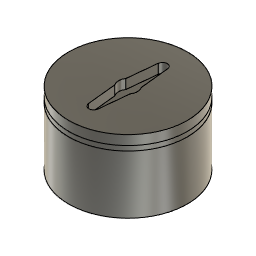
servo_double v2 (Autodesk Fusion 360 archive; units mm, degrees)
design "servo"
Autodesk Fusion 360 part; units mm, degrees
sketch "スケッチ1" plane through (0, 0, 0) normal (0, 0, 1) x (1, 0, 0)
  circle A0 centre (0, 0) radius 25
  line L0 (3.2646, -2.3114) -> (1.9895, -14.7047)
  line L1 (-3.2646, -2.3114) -> (-1.9895, -14.7047)
  line L2 (-3.2597, 2.3182) -> (-1.9896, 14.704)
  arc A1 (1.9896, 14.704) -> (-1.9896, 14.704) centre (0, 14.5) ccw
  arc A2 (-1.9895, -14.7047) -> (1.9895, -14.7047) centre (0, -14.5) ccw
  line L3 (3.2597, 2.3182) -> (1.9896, 14.704)
  arc A3 (3.2646, -2.3114) -> (3.2597, 2.3182) centre (0, 0) ccw
  arc A4 (-3.2597, 2.3182) -> (-3.2646, -2.3114) centre (0, 0) ccw
  dimension "d1" = 50
  dimension "d3" = 4
  dimension "d5" = 4
  dimension "d7" = 8
  constraint coincident A0.centre A3.centre
  constraint tangent L0 A2
  constraint tangent L1 A2
  constraint tangent L2 A1
  constraint coincident L2.start A3
  constraint concentric A3 A4
  measures "d1" diameter of A0
  measures "d3" diameter of A1
  measures "d5" diameter of A2
  measures "d7" diameter of A3
extrude "押し出し1" add sketch "スケッチ1" along normal blind 4 makes body 1
sketch "スケッチ2" plane through (0, 0, 4) normal (0, 0, 1) x (-1, 0, 0)
  arc A0 (-3.2646, 2.3114) -> (-3.2597, -2.3182) centre (0, 0) ccw
  line L0 (-3.2646, 2.3114) -> (-1.9895, 14.7047)
  arc A1 (1.9895, 14.7047) -> (-1.9895, 14.7047) centre (0, 14.5) ccw
  line L1 (1.9895, 14.7047) -> (3.2646, 2.3114)
  arc A2 (3.2597, -2.3182) -> (3.2646, 2.3114) centre (0, 0) ccw
  line L2 (3.2597, -2.3182) -> (1.9896, -14.704)
  arc A3 (-1.9896, -14.704) -> (1.9896, -14.704) centre (0, -14.5) ccw
  line L3 (-1.9896, -14.704) -> (-3.2597, -2.3182)
  circle A4 centre (0, 0) radius 25
  circle A5 centre (55, 0) radius 25
  dimension "d10" = 50
  measures "d10" diameter of A5
extrude "押し出し2" add sketch "スケッチ2" along normal blind 2 separate body contours A5 makes body 2
move_body "移動1" bodies 2 to x (1, 0, 0) y (0, 1, 0) z (0, 0, 1) at (55, 0, -6)
extrude "押し出し3" cut 1 faces at (-7.8601, -11.3401, 4) along direction (0, 0, -1) blind 1 on bodies 1 bodies 1
sketch "スケッチ3" plane through (0, 0, 3) normal (0, 0, 1) x (-1, 0, 0)
  arc A0 (-3.2646, 2.3114) -> (-3.2597, -2.3182) centre (0, 0) ccw
  line L0 (-3.2646, 2.3114) -> (-1.9895, 14.7047)
  arc A1 (1.9895, 14.7047) -> (-1.9895, 14.7047) centre (0, 14.5) ccw
  line L1 (1.9895, 14.7047) -> (3.2646, 2.3114)
  arc A2 (3.2597, -2.3182) -> (3.2646, 2.3114) centre (0, 0) ccw
  line L2 (3.2597, -2.3182) -> (1.9896, -14.704)
  arc A3 (-1.9896, -14.704) -> (1.9896, -14.704) centre (0, -14.5) ccw
  line L3 (-1.9896, -14.704) -> (-3.2597, -2.3182)
  circle A4 centre (0, 0) radius 25
  circle A5 centre (-74.9851, 0.0123) radius 25
  line L4 (-97.2842, -2.9877) -> (-80.9851, -2.9877)
  line L5 (-77.9851, -5.9877) -> (-77.9851, -22.2869)
  line L6 (-52.686, 3.0123) -> (-68.9851, 3.0123)
  line L7 (-71.9851, 6.0123) -> (-71.9851, 22.3114)
  arc A6 (-77.9851, -5.9877) -> (-80.9851, -2.9877) centre (-80.9851, -5.9877) ccw
  arc A7 (-71.9851, 6.0123) -> (-68.9851, 3.0123) centre (-68.9851, 6.0123) ccw
  arc A8 (-77.9851, -22.2869) -> (-52.686, 3.0123) centre (-74.9851, 0.0123) ccw
  arc A9 (-71.9851, 22.3114) -> (-97.2842, -2.9877) centre (-74.9851, 0.0123) ccw
  dimension "d15" = 50
  dimension "d16" = 45
  dimension "d19" = 6
  dimension "d20" = 6
  dimension "d21" = 3
  dimension "d22" = 3
  dimension "d23" = 3
  dimension "d24" = 3
  constraint concentric A5 A8
  constraint horizontal L4
  constraint vertical L5
  constraint horizontal L6
  constraint vertical L7
  constraint tangent L5 A6
  constraint tangent L4 A6
  constraint tangent L6 A7
  constraint tangent L7 A7
  constraint concentric A8 A9
  measures "d15" diameter of A5
  measures "d16" diameter of A8
  measures "d19" distance of L4 L6
  measures "d20" distance of L5 L7
  measures "d21" distance of A5.centre L4
  measures "d22" distance of A5.centre L5
  measures "d23" radius of A6
  measures "d24" radius of A7
extrude "押し出し4" add sketch "スケッチ3" along normal blind 10 separate body contours A5 makes body 3
extrude "押し出し5" add 1 faces at (-7.8601, -11.3401, 3) along direction (0, 0, 1) blind 1 on bodies 1 bodies 1
move_body "移動2" bodies 1 2 to x (1, 0, 0) y (0, 1, 0) z (0, 0, 1) at (75, 0, 15)
move_body "移動3" bodies 3 1 2 to x (1, 0, 0) y (0, 1, 0) z (0, 0, 1) at (-75, 0, 0)
sketch "スケッチ4" plane through (0, 0, 3) normal (0, 0, -1) x (1, 0, 0)
  line L0 (-3.0149, 6.0123) -> (-3.0149, 22.3114)
  arc A0 (22.2842, -2.9877) -> (-3.0149, 22.3114) centre (-0.0149, 0.0123) ccw
  line L1 (22.2842, -2.9877) -> (5.9851, -2.9877)
  arc A1 (5.9851, -2.9877) -> (2.9851, -5.9877) centre (5.9851, -5.9877) ccw
  line L2 (2.9851, -5.9877) -> (2.9851, -22.2869)
  arc A2 (-22.314, 3.0123) -> (2.9851, -22.2869) centre (-0.0149, 0.0123) ccw
  line L3 (-22.314, 3.0123) -> (-6.0149, 3.0123)
  arc A3 (-6.0149, 3.0123) -> (-3.0149, 6.0123) centre (-6.0149, 6.0123) ccw
  circle A4 centre (-0.0149, 0.0123) radius 25
  circle A5 centre (-0.0149, 0.0123) radius 25
  circle A6 centre (-0.0149, 0.0123) radius 22.5
  dimension "d29" = 50
  dimension "d30" = 45
  constraint concentric A0 A5
  constraint concentric A5 A6
  measures "d29" diameter of A5
  measures "d30" diameter of A6
extrude "押し出し6" add sketch "スケッチ4" along normal blind 15 bodies 3
move_body "移動4" bodies 1 2 3 to x (1, 0, 0) y (0, 1, 0) z (0, 0, 1) at (0, 0, 12)
sketch "スケッチ5" plane through (0, 0, 0) normal (0, 1, 0) x (1, 0, 0)
extrude "押し出し7" cut 1 faces at (-3.606, 23.839, 0) along direction (0, 0, 1) blind 0.5 on bodies 3 bodies 3

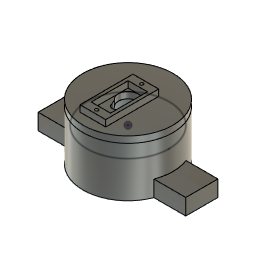
design "servo_up"
Autodesk Fusion 360 part; units mm, degrees
sketch "スケッチ1" plane through (0, 0, 0) normal (0, 0, 1) x (1, 0, 0)
  circle A0 centre (0, 0) radius 25.5
  circle A1 centre (0, 0) radius 22.5
  circle A2 centre (0, 0) radius 28
  dimension "d1" = 51
  dimension "d2" = 45
  dimension "d3" = 56
  constraint coincident A0.centre A1.centre
  constraint concentric A0 A2
  measures "d1" diameter of A0
  measures "d2" diameter of A1
  measures "d3" diameter of A2
extrude "押し出し1" add sketch "スケッチ1" along normal blind 25 contours A2 makes body 1
sketch "スケッチ2" plane through (0, 0, 0) normal (0, 0, 1) x (1, 0, 0)
  circle A0 centre (0, 0) radius 22.5
  circle A1 centre (0, 0) radius 25.5
  dimension "d6" = 45
  dimension "d7" = 51
  constraint coincident A0.centre A1.centre
  measures "d6" diameter of A0
  measures "d7" diameter of A1
extrude "押し出し2" add sketch "スケッチ2" along normal blind 15 bodies 1
sketch "スケッチ3" plane through (0, 0, 0) normal (0, 0, 1) x (1, 0, 0)
  line L0 (-31.9093, 14.985) -> (-51.9093, 14.985)
  line L1 (-51.9093, 14.985) -> (-51.9093, -15.015)
  line L2 (-51.9093, -15.015) -> (-31.9093, -15.015)
  line L3 (-31.9093, -15.015) -> (-31.9093, 14.985)
  circle A0 centre (-41.9093, -0.0927) radius 7
  dimension "d10" = 20
  dimension "d11" = 30
  dimension "d12" = 14
  dimension "d13" = 10
  constraint horizontal L0
  constraint vertical L1
  constraint horizontal L2
  constraint vertical L3
  measures "d10" distance of L0.start L0.end
  measures "d11" distance of L0.end L1.end
  measures "d12" diameter of A0
  measures "d13" distance of L1 A0.centre
sketch "スケッチ4" plane through (0, 0, 0) normal (0, 0, 1) x (1, 0, 0)
sketch "スケッチ5" plane through (0, 0, 0) normal (0, 1, 0) x (1, 0, 0)
sketch "スケッチ6" plane through (0, 0, 0) normal (0, 0, 1) x (1, 0, 0)
  line L0 (-60, 20) -> (-40, 20)
  line L1 (-40, 20) -> (-40, 0)
  line L2 (-40, 0) -> (-60, 0)
  line L3 (-60, 0) -> (-60, 20)
  dimension "d16" = 20
  constraint horizontal L0
  constraint vertical L1
  constraint horizontal L2
  constraint vertical L3
  measures "d16" distance of L0.start L0.end
extrude "押し出し4" add sketch "スケッチ6" along normal blind 10 separate body makes body 2
sketch "スケッチ7" plane through (0, 0, 0) normal (0, 0, 1) x (1, 0, 0)
  circle A0 centre (-50, 10) radius 7
  dimension "d19" = 14
  measures "d19" diameter of A0
extrude "押し出し5" cut sketch "スケッチ7" along normal blind 2.5 bodies 2
copy_body "ボディのコピーと貼り付け1" bodies 2 makes body 3
sketch "スケッチ8" plane through (0, 0, 0) normal (0, 0, 1) x (1, 0, 0)
  line L0 (35, 20) -> (55, 20)
  line L1 (55, 20) -> (55, 0)
  line L2 (55, 0) -> (35, 0)
  line L3 (35, 0) -> (35, 20)
  dimension "d22" = 20
  constraint horizontal L0
  constraint vertical L1
  constraint horizontal L2
  constraint vertical L3
  measures "d22" distance of L0.start L0.end
extrude "押し出し6" add sketch "スケッチ8" along normal blind 10 separate body makes body 4
sketch "スケッチ9" plane through (0, 0, 0) normal (0, 0, 1) x (1, 0, 0)
  circle A0 centre (45, 10) radius 7
  dimension "d25" = 14
  measures "d25" diameter of A0
extrude "押し出し7" cut sketch "スケッチ9" along normal blind 2.5 bodies 4
move_body "移動1" bodies 3 2 to x (1, 0, 0) y (0, 1, 0) z (0, 0, 1) at (0, -20, 0)
move_face "面を移動1" by (0, 10, 0) 1 faces at (-53.3333, -6.6667, 10) on bodies 3
move_body "移動2" bodies 2 3 to x (1, 0, 0) y (0, 1, 0) z (0, 0, 1) at (0, 10, 0)
move_body "移動3" bodies 2 3 to x (1, 0, 0) y (0, 1, 0) z (0, 0, 1) at (14, 0, 0)
move_body "移動4" bodies 4 to x (1, 0, 0) y (0, 1, 0) z (0, 0, 1) at (-9, -10, 0)
sketch "スケッチ10" plane through (0, 0, 0) normal (0, 0, 1) x (1, 0, 0)
  line L0 (70, 15) -> (140, 15)
  line L1 (140, 15) -> (140, -23)
  line L2 (140, -23) -> (70, -23)
  line L3 (70, -23) -> (70, 15)
  line L4 (90, 0) -> (113, 0)
  line L5 (113, 0) -> (113, -12)
  line L6 (113, -12) -> (90, -12)
  line L7 (90, -12) -> (90, 0)
  dimension "d28" = 70
  dimension "d29" = 23
  dimension "d30" = 12
  dimension "d31" = 38
  constraint horizontal L0
  constraint vertical L1
  constraint horizontal L2
  constraint vertical L3
  constraint horizontal L4
  constraint vertical L5
  constraint horizontal L6
  constraint vertical L7
  measures "d28" distance of L0.start L0.end
  measures "d29" distance of L4.start L4.end
  measures "d30" distance of L4 L6
  measures "d31" distance of L0.end L1.end
sketch "スケッチ11" plane through (0, 0, 0) normal (0, 0, 1) x (1, 0, 0)
  line L0 (113, -12) -> (118, -12)
  line L1 (118, -12) -> (118, 0)
  line L2 (118, 0) -> (113, 0)
  line L3 (113, 0) -> (113, -12)
  line L4 (90, -12) -> (85, -12)
  line L5 (85, -12) -> (85, 0)
  line L6 (85, 0) -> (90, 0)
  line L7 (90, 0) -> (90, -12)
  dimension "d34" = 5
  dimension "d35" = 5
  dimension "d36" = 12
  dimension "d37" = 12
  constraint horizontal L0
  constraint vertical L1
  constraint horizontal L2
  constraint vertical L3
  constraint horizontal L4
  constraint vertical L5
  constraint horizontal L6
  constraint vertical L7
  measures "d34" distance of L0.start L0.end
  measures "d35" distance of L4.start L4.end
  measures "d36" distance of L0 L2
  measures "d37" distance of L4 L6
sketch "スケッチ12" plane through (0, 0, 0) normal (0, 0, 1) x (1, 0, 0)
  circle A0 centre (-102, 0) radius 28
  line L0 (-99.5001, -7.5215) -> (-99.4823, -5.4462)
  line L1 (-104.5, -7.5) -> (-104.5, -5.4544)
  arc A1 (-104.5, -7.5) -> (-99.5001, -7.5215) centre (-102, -7.5) ccw
  arc A2 (-99.4823, -5.4462) -> (-104.5, -5.4544) centre (-102, 0) ccw
  dimension "d40" = 56
  dimension "d41" = 12
  dimension "d42" = 5
  dimension "d43" = 7.5
  constraint concentric A0 A2
  constraint tangent L0 A1
  constraint tangent L1 A1
  constraint vertical L1
  measures "d40" diameter of A0
  measures "d41" diameter of A2
  measures "d42" diameter of A1
  measures "d43" distance of A0.centre A1.centre
extrude "押し出し10" add sketch "スケッチ12" along normal blind 5 separate body makes body 5
sketch "スケッチ13" plane through (0, 0, 15) normal (0, 0, 1) x (-1, 0, 0)
  circle A0 centre (0, 0) radius 22.5
  circle A1 centre (0, 0) radius 25.5
sketch "スケッチ14" plane through (0, 0, 15) normal (0, 0, 1) x (1, 0, 0)
  circle A0 centre (0, 0) radius 25.5
  dimension "d46" = 51
  constraint coincident A0.centre origin
  measures "d46" diameter of A0
sketch "スケッチ15" plane through (0, 0, 15) normal (0, 0, 1) x (1, 0, 0)
sketch "スケッチ16" plane through (0, 0, 15) normal (0, 0, 1) x (1, 0, 0)
  line L0 (-108, 6.0876) -> (-96, 6.0876)
  line L1 (-96, 6.0876) -> (-96, -16.9124)
  line L2 (-96, -16.9124) -> (-108, -16.9124)
  line L3 (-108, -16.9124) -> (-108, 6.0876)
  line L4 (-110, 11.0876) -> (-94, 11.0876)
  line L5 (-94, 11.0876) -> (-94, -21.9124)
  line L6 (-94, -21.9124) -> (-110, -21.9124)
  line L7 (-110, -21.9124) -> (-110, 11.0876)
  dimension "d47" = 12
  dimension "d48" = 23
  dimension "d50" = 5
  dimension "d51" = 5
  dimension "d52" = 2
  dimension "d53" = 2
  constraint horizontal L0
  constraint vertical L1
  constraint horizontal L2
  constraint vertical L3
  constraint horizontal L4
  constraint vertical L5
  constraint horizontal L6
  constraint vertical L7
  measures "d47" distance of L1 L3
  measures "d48" distance of L0 L2
  measures "d50" distance of L2 L6
  measures "d51" distance of L0 L4
  measures "d52" distance of L1 L5
  measures "d53" distance of L3 L7
extrude "押し出し11" add sketch "スケッチ16" along normal blind 7 separate body makes body 6
move_body "移動5" bodies 6 to x (1, 0, 0) y (0, 1, 0) z (0, 0, 1) at (0, 0, -10)
extrude "押し出し12" cut 1 faces at (-92.8319, -10.3859, 0) along direction (0, 0, 1) blind 1 on bodies 5 bodies 5
extrude "押し出し13" cut sketch "スケッチ13" against normal blind 15 bodies 1
move_body "移動6" bodies 6 5 to x (1, 0, 0) y (0, 1, 0) z (0, 0, 1) at (0, 0, -1)
move_body "移動7" bodies 5 6 to x (1, 0, 0) y (0, 1, 0) z (0, 0, 1) at (102, 0, 25)
sketch "スケッチ17" plane through (0, 0, 0) normal (0, 1, 0) x (1, 0, 0)
sketch "スケッチ18" plane through (0, 0, 29) normal (0, 0, 1) x (-1, 0, 0)
  arc A0 (2.5, 7.5) -> (-2.4999, 7.5215) centre (0, 7.5) ccw
  line L0 (2.5, 7.5) -> (2.5, 5.4544)
  arc A1 (-2.5177, 5.4462) -> (2.5, 5.4544) centre (0, 0) ccw
  line L1 (-2.5177, 5.4462) -> (-2.4999, 7.5215)
  circle A2 centre (0, 0) radius 28
  line L2 (3.863, 4.591) -> (2.5, 7.5)
  line L3 (-3.873, 4.5826) -> (-2.4999, 7.5215)
  constraint coincident A0.start L0.start
  constraint coincident A0.end L1.end
  constraint coincident A1 L2.start
  constraint coincident A1 L3.start
sketch "スケッチ19" plane through (0, 0, 36) normal (0, 0, 1) x (-1, 0, 0)
  line L0 (-6, 16.9124) -> (6, 16.9124)
  line L1 (6, 16.9124) -> (6, -6.0876)
  line L2 (6, -6.0876) -> (-6, -6.0876)
  line L3 (-6, -6.0876) -> (-6, 16.9124)
  line L4 (8, 21.9124) -> (-8, 21.9124)
  line L5 (-8, 21.9124) -> (-8, -11.0876)
  line L6 (-8, -11.0876) -> (8, -11.0876)
  line L7 (8, -11.0876) -> (8, 21.9124)
  circle A0 centre (0.0951, 19.4124) radius 1
  circle A1 centre (0, -8.5876) radius 1
  dimension "d60" = 2
  dimension "d61" = 2.5
  dimension "d62" = 2
  dimension "d63" = 2.5
  measures "d60" diameter of A0
  measures "d61" distance of L0 A0.centre
  measures "d62" diameter of A1
  measures "d63" distance of L6 A1.centre
extrude "押し出し14" cut sketch "スケッチ19" against normal blind 5 contours A0 | A1 bodies 6
extrude "押し出し15" cut 1 faces at (4.9646, -19.4621, 36) along direction (0, 0, -1) blind 3 on bodies 6 bodies 6
extrude "押し出し16" cut 1 faces at (0.0742, 8.2626, 31) along direction (0, 0, -1) blind 3 on bodies 6 bodies 5 6
extrude "押し出し17" cut 1 faces at (-0.3029, -19.673, 31) along direction (0, 0, -1) blind 3 on bodies 6 bodies 5 6
extrude "押し出し18" cut sketch "スケッチ18" against normal blind 4 contours L0 A1 L2 | A1 L1 L3 bodies 5
extrude "押し出し19" add 1 faces at (26.9675, -2.6579, 0) along direction (0, 0, -1) blind 5 on bodies 1 bodies 1 2 3 4
extrude "押し出し20" add 1 faces at (26.9675, -2.6579, -5) along direction (0, 0, -1) blind 1 on bodies 1 bodies 1
move_face "面を移動2" to x (1, 0, 0) y (0, 1, 0) z (0, 0, 1) at (0, 0, -6) 6 faces at (36.2255, -8.9935, 0) (42.9913, -0.3489, 1.6667) (37.1973, 2.224, 2.5) (40, 0, 10) (39.3845, 10, 6.6667) (46, 3.3333, 3.3333) on bodies 1
move_face "面を移動3" to x (1, 0, 0) y (0, 1, 0) z (0, 0, 1) at (0, 0, -6) 7 faces at (-34.8027, 2.224, 2.5) (-29.0087, -0.3489, 1.6667) (-36.2255, -8.9935, 0) (-46, -3.3333, 3.3333) (-32.7689, 10, 6.6667) (-39.9751, -0.6811, 10) (-32.7689, -10, 6.6667) on bodies 1
sketch "スケッチ20" plane through (0, 0, -6) normal (0, 0, -1) x (1, 0, 0)
  circle A0 centre (-36, 0) radius 7
  circle A1 centre (0, 0) radius 25.5
  line L0 (26.1534, -10) -> (46, -10)
  line L1 (46, -10) -> (46, 10)
  line L2 (46, 10) -> (26.1534, 10)
  arc A2 (26.1534, 10) -> (-26.1534, 10) centre (0, 0) ccw
  line L3 (-26.1534, 10) -> (-46, 10)
  line L4 (-46, 10) -> (-46, -10)
  line L5 (-46, -10) -> (-26.1534, -10)
  arc A3 (-26.1534, -10) -> (26.1534, -10) centre (0, 0) ccw
  circle A4 centre (36, 0) radius 7
sketch "スケッチ21" plane through (0, 0, 0) normal (0, 1, 0) x (1, 0, 0)
